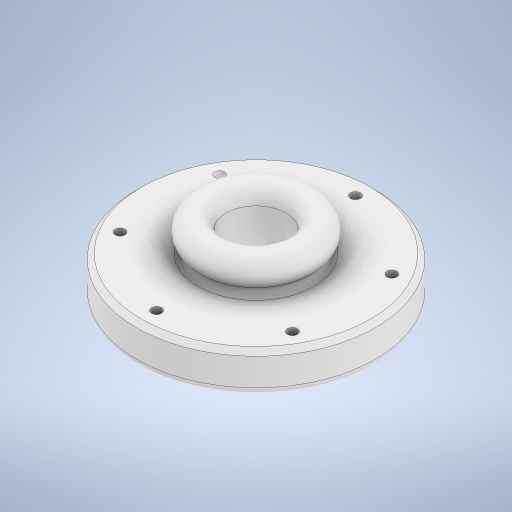
# Autodesk Inventor part: Bottom
Saved by Autodesk Inventor 2023 (Build 270158030, 158C)
## iProperties
Created: 2022-09-15
Part Number: Bottom
Material: ABS Plastic
Document SubType Name: Modeling
Designer: cjj5381
Density: 1.06 g/cm^3
Appearance: Smooth - White
Author: cjj5381
Autodesk Inventor part; units mm, degrees
ref_plane "YZ Plane" through (0, 0, 0) normal (1, 0, 0) x (0, 1, 0)
ref_plane "XZ Plane" through (0, 0, 0) normal (0, 1, 0) x (-1, 0, 0)
ref_plane "XY Plane" through (0, 0, 0) normal (0, 0, 1) x (1, 0, 0)
sketch "Sketch1" plane through (0, 0, 0) normal (0, 1, 0) x (-1, 0, 0)
  circle A0 centre (0, 0) radius 76.2
  dimension "d0" = 152.4
  constraints: 1 centre point, 1 coincident
  measures "d0" diameter of A0
extrude "Main-Body" add sketch "Sketch1" along normal blind 25.4
sketch "Sketch3" plane through (0, 0, 0) normal (0, 0, 1) x (1, 0, 0)
  line L0 (0, 25.4) -> (19.05, 25.4)
  line L1 (19.05, 25.4) -> (19.05, 12.7)
  line L2 (76.2, 25.4) -> (-76.2, 25.4) projected
  arc A0 (19.05, 12.7) -> (31.75, 0) centre (31.75, 12.7) ccw
  line L3 (76.2, 0) -> (-76.2, 0) projected
  line L4 (31.75, 0) -> (0, 0)
  line L5 (0, 0) -> (0, 25.4)
  dimension "d12" = 25.4
  dimension "d19" = 19.05
  constraints: 8 end point, 3 tangent, 2 collinear, 2 point on circle, 2 vertical, 1 centre point, 1 horizontal, 1 point on line
  measures "d12" diameter of A0
  measures "d19" distance of L0.start L0.end
revolve "Middle-Cutout" cut sketch "Sketch3" angle 360 about axis through (0, 0, 0) along (0, 1, 0)
sketch "Sketch4" plane through (0, 0, 0) normal (0, 0, 1) x (1, 0, 0)
  line L0 (19.05, 25.4) -> (19.05, 12.7) projected
  line L1 (0, 0) -> (0, 33.6646)
  arc A0 (34.8752, 30.9563) -> (19.05, 38.1) centre (28.575, 38.1) ccw
  arc A1 (34.8752, 30.9563) -> (36.9753, 25.4) centre (36.9753, 28.575) ccw
  line L2 (76.2, 25.4) -> (-76.2, 25.4) projected
  line L3 (19.05, 25.4) -> (19.05, 38.1)
  line L4 (36.9753, 25.4) -> (19.05, 25.4)
  dimension "d48" = 9.525
  dimension "d50" = 12.7
  dimension "d51" = 3.175
  constraints: 6 end point, 4 point on circle, 3 tangent, 2 centre point, 1 perpendicular, 1 point on line, 1 vertical
  measures "d48" radius of A0
  measures "d50" distance from line of L2 A0.centre
  measures "d51" radius of A1
revolve "Bump" add sketch "Sketch4" angle 360 about axis through (0, 0, 0) along (0, 1, 0)
fillet "Fillet4" radius 4.7625 1 edges at (76.2, 0, 0)
sketch "Sketch6" plane through (0, 25.4, 0) normal (0, 1, 0) x (1, 0, 0)
  line L0 (0, 0) -> (0, -63.5)
  point P0 (0, -63.5)
  dimension "d41" = 63.5
  constraints: 2 end point, 1 coincident, 1 vertical
  measures "d41" distance of L0.start L0.end
hole "Hole1" at (0, 25.4, 63.5) direction (0, -1, 0) diameter 6.4 depth 10.6
pattern_circular "Circular Pattern1" count 6 over 360 about axis through (0, 19.05, 0) along (0, -1, 0) of "Hole1"
chamfer "Chamfer1" distance 3.175 angle 45 1 edges at (76.2, 25.4, 0)
body "Solid1"
